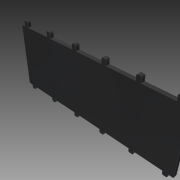
# Autodesk Inventor part: spool_stand_brace_bottom
Saved by Autodesk Inventor 2014 (Build 180170000, 170)
## iProperties
Created: 2014-04-08
Part Number: spool_stand_brace_bottom
Material: Plywood, Finish
Document SubType Name: Modeling
Designer: buben
Density: 0.552 g/cm^3
Appearance: Anodized - Dark Gray
Author: buben
Autodesk Inventor part; units mm, degrees
ref_plane "YZ Plane" through (0, 0, 0) normal (1, 0, 0) x (0, 1, 0)
ref_plane "XZ Plane" through (0, 0, 0) normal (0, 1, 0) x (-1, 0, 0)
ref_plane "XY Plane" through (0, 0, 0) normal (0, 0, 1) x (1, 0, 0)
sketch "Sketch1" plane through (0, 0, 0) normal (0, 1, 0) x (-1, 0, 0)
  line L0 (0, 0) -> (-296, 0)
  line L1 (-296, 0) -> (-296, -110)
  line L2 (-296, -110) -> (0, -110)
  line L3 (0, -110) -> (0, 0)
  dimension "d0" = 296
  dimension "d1" = 110
  constraints: 8 end point, 2 parallel, 1 horizontal, 1 perpendicular
  measures "d0" distance of L0.start L0.end
  measures "d1" distance of L2.end L0.start
extrude "Extrusion1" add sketch "Sketch1" along normal blind 6.5
sketch "Sketch2" plane through (0, 6.5, 0) normal (0, 1, 0) x (1, 0, 0)
  line L0 (296, 0) -> (296, 110) projected
  line L1 (296, 110) -> (0, 110) projected
  line L2 (0, 110) -> (0, 0) projected
  line L3 (8, 110) -> (16, 110)
  line L4 (16, 110) -> (16, 114.5)
  line L5 (14, 116.5) -> (10, 116.5)
  line L6 (8, 114.5) -> (8, 110)
  line L7 (62.4, 110) -> (70.4, 110)
  line L8 (70.4, 110) -> (70.4, 114.5)
  line L9 (68.4, 116.5) -> (64.4, 116.5)
  line L10 (62.4, 114.5) -> (62.4, 110)
  line L11 (116.8, 110) -> (124.8, 110)
  line L12 (124.8, 110) -> (124.8, 114.5)
  line L13 (122.8, 116.5) -> (118.8, 116.5)
  line L14 (116.8, 114.5) -> (116.8, 110)
  line L15 (171.2, 110) -> (179.2, 110)
  line L16 (179.2, 110) -> (179.2, 114.5)
  line L17 (177.2, 116.5) -> (173.2, 116.5)
  line L18 (171.2, 114.5) -> (171.2, 110)
  line L19 (225.6, 110) -> (233.6, 110)
  line L20 (233.6, 110) -> (233.6, 114.5)
  line L21 (231.6, 116.5) -> (227.6, 116.5)
  line L22 (225.6, 114.5) -> (225.6, 110)
  line L23 (280, 110) -> (288, 110)
  line L24 (288, 110) -> (288, 114.5)
  line L25 (286, 116.5) -> (282, 116.5)
  line L26 (280, 114.5) -> (280, 110)
  arc A0 (10, 116.5) -> (8, 114.5) centre (10, 114.5) ccw
  arc A1 (16, 114.5) -> (14, 116.5) centre (14, 114.5) ccw
  arc A2 (64.4, 116.5) -> (62.4, 114.5) centre (64.4, 114.5) ccw
  arc A3 (70.4, 114.5) -> (68.4, 116.5) centre (68.4, 114.5) ccw
  arc A4 (118.8, 116.5) -> (116.8, 114.5) centre (118.8, 114.5) ccw
  arc A5 (124.8, 114.5) -> (122.8, 116.5) centre (122.8, 114.5) ccw
  arc A6 (173.2, 116.5) -> (171.2, 114.5) centre (173.2, 114.5) ccw
  arc A7 (179.2, 114.5) -> (177.2, 116.5) centre (177.2, 114.5) ccw
  arc A8 (227.6, 116.5) -> (225.6, 114.5) centre (227.6, 114.5) ccw
  arc A9 (233.6, 114.5) -> (231.6, 116.5) centre (231.6, 114.5) ccw
  arc A10 (282, 116.5) -> (280, 114.5) centre (282, 114.5) ccw
  arc A11 (288, 114.5) -> (286, 116.5) centre (286, 114.5) ccw
  line L27 (16, 112.25) -> (62.4, 112.25) construction
  line L28 (70.4, 112.25) -> (116.8, 112.25) construction
  line L29 (124.8, 112.25) -> (171.2, 112.25) construction
  line L30 (179.2, 112.25) -> (225.6, 112.25) construction
  line L31 (233.6, 112.25) -> (280, 112.25) construction
  line L32 (0, 55) -> (296, 55) construction
  line L33 (0, 0) -> (296, 0) projected
  line L34 (296, 0) -> (296, 110) projected
  line L35 (296, 110) -> (0, 110) projected
  line L36 (0, 110) -> (0, 0) projected
  line L37 (8, 0) -> (16, 0)
  line L38 (16, 0) -> (16, -7.5)
  line L39 (14, -9.5) -> (10, -9.5)
  line L40 (8, -7.5) -> (8, 0)
  line L41 (62.4, 0) -> (70.4, 0)
  line L42 (70.4, 0) -> (70.4, -7.5)
  line L43 (68.4, -9.5) -> (64.4, -9.5)
  line L44 (62.4, -7.5) -> (62.4, 0)
  line L45 (116.8, 0) -> (124.8, 0)
  line L46 (124.8, 0) -> (124.8, -7.5)
  line L47 (122.8, -9.5) -> (118.8, -9.5)
  line L48 (116.8, -7.5) -> (116.8, 0)
  line L49 (171.2, 0) -> (179.2, 0)
  line L50 (179.2, 0) -> (179.2, -7.5)
  line L51 (177.2, -9.5) -> (173.2, -9.5)
  line L52 (171.2, -7.5) -> (171.2, 0)
  line L53 (225.6, 0) -> (233.6, 0)
  line L54 (233.6, 0) -> (233.6, -7.5)
  line L55 (231.6, -9.5) -> (227.6, -9.5)
  line L56 (225.6, -7.5) -> (225.6, 0)
  line L57 (280, 0) -> (288, 0)
  line L58 (288, 0) -> (288, -7.5)
  line L59 (286, -9.5) -> (282, -9.5)
  line L60 (280, -7.5) -> (280, 0)
  arc A12 (8, -7.5) -> (10, -9.5) centre (10, -7.5) ccw
  arc A13 (14, -9.5) -> (16, -7.5) centre (14, -7.5) ccw
  arc A14 (62.4, -7.5) -> (64.4, -9.5) centre (64.4, -7.5) ccw
  arc A15 (68.4, -9.5) -> (70.4, -7.5) centre (68.4, -7.5) ccw
  arc A16 (116.8, -7.5) -> (118.8, -9.5) centre (118.8, -7.5) ccw
  arc A17 (122.8, -9.5) -> (124.8, -7.5) centre (122.8, -7.5) ccw
  arc A18 (171.2, -7.5) -> (173.2, -9.5) centre (173.2, -7.5) ccw
  arc A19 (177.2, -9.5) -> (179.2, -7.5) centre (177.2, -7.5) ccw
  arc A20 (225.6, -7.5) -> (227.6, -9.5) centre (227.6, -7.5) ccw
  arc A21 (231.6, -9.5) -> (233.6, -7.5) centre (231.6, -7.5) ccw
  arc A22 (280, -7.5) -> (282, -9.5) centre (282, -7.5) ccw
  arc A23 (286, -9.5) -> (288, -7.5) centre (286, -7.5) ccw
  dimension "d4" = 2
  dimension "d5" = 8
  dimension "d6" = 8
  dimension "d7" = 8
  dimension "d8" = 8
  dimension "d9" = 8
  dimension "d10" = 8
  dimension "d11" = 6.5
  dimension "d12" = 8
  dimension "d13" = 8
  dimension "d16" = 2
  dimension "d17" = 9.5
  constraints: 108 end point, 48 point on circle, 48 tangent, 26 collinear, 24 centre point, 24 parallel, 22 equal radius, 12 horizontal, 12 midpoint, 12 perpendicular, 12 point on line
  measures "d4" radius of A0
  measures "d5" distance between parallel lines of L6 L4
  measures "d6" distance between parallel lines of L8 L10
  measures "d7" distance between parallel lines of L12 L14
  measures "d8" distance between parallel lines of L16 L18
  measures "d9" distance between parallel lines of L20 L22
  measures "d10" distance between parallel lines of L24 L26
  measures "d11" distance between parallel lines of L3 L5
  measures "d12" distance between parallel lines of L2 L6
  measures "d13" distance between parallel lines of L0 L24
  measures "d16" radius of A12
  measures "d17" distance between parallel lines of L33 L39
extrude "Extrusion3" add sketch "Sketch2" against normal blind 6.5 contours L58 A23 L59 A22 L60 L33 | L1 L26 A10 L25 A11 L24 | L54 A21 L55 A20 L56 L33 | L1 L22 A8 L21 A9 L20 | L50 A19 L51 A18 L52 L33 | L1 L18 A6 L17 A7 L16 | L46 A17 L47 A16 L48 L33 | L1 L14 A4 L13 A5 L12 | L42 A15 L43 A14 L44 L33 | L1 L10 A2 L9 A3 L8 | L38 A13 L39 A12 L40 L33 | L1 L6 A0 L5 A1 L4
equation "\"d6\" = d5"
equation "\"d7\" = d6"
equation "\"d8\" = d7"
equation "\"d9\" = d8"
equation "\"d10\" = d9"
equation "\"d13\" = d12"
body "Solid1"
